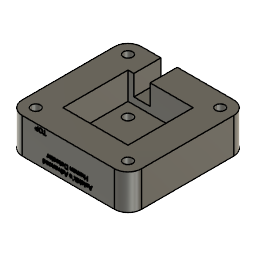
Sensor_Bottom (Autodesk Fusion 360 design; units mm, degrees)
part number: 2026-02-06-21-46-18-488
Autodesk Fusion 360 part; units mm, degrees
sketch "Sketch1" plane through (0, 0, 0) normal (0, 0, 1) x (1, 0, 0)
  line L0 (39, 33) -> (15, 33)
  line L1 (15, 33) -> (15, 9)
  line L2 (15, 9) -> (39, 9)
  line L3 (39, 9) -> (39, 33)
  circle A0 centre (44, 38) radius 1.7
  circle A1 centre (10, 38) radius 1.7
  circle A2 centre (44, 4) radius 1.7
  circle A3 centre (10, 4) radius 1.7
  line L4 (49, 43) -> (5, 43)
  line L5 (5, 43) -> (5, -1)
  line L6 (5, -1) -> (49, -1)
  line L7 (49, -1) -> (49, 43)
  circle A4 centre (44, 4) radius 3
  circle A5 centre (10, 4) radius 3
  circle A6 centre (44, 38) radius 3
  circle A7 centre (10, 38) radius 3
  dimension "d1" = 24
  dimension "d2" = 24
  dimension "d7" = 3.4
  dimension "d8" = 3.4
  dimension "d9" = 3.4
  dimension "d10" = 3.4
  dimension "d11" = 44
  dimension "d12" = 44
  dimension "d13" = 10
  dimension "d14" = 10
  dimension "d15" = 5
  dimension "d16" = 5
  dimension "d17" = 5
  dimension "d18" = 5
  dimension "d19" = 5
  dimension "d20" = 5
  dimension "d21" = 5
  dimension "d22" = 5
  dimension "d23" = 6
  dimension "d24" = 6
  dimension "d25" = 6
  dimension "d26" = 6
  constraint horizontal L0
  constraint vertical L1
  constraint horizontal L2
  constraint vertical L3
  constraint horizontal L4
  constraint vertical L5
  constraint horizontal L6
  constraint vertical L7
  constraint concentric A2 A4
  constraint concentric A3 A5
  constraint concentric A0 A6
  constraint concentric A1 A7
  measures "d1" distance of L0.start L0.end
  measures "d2" distance of L0.start L2.end
  measures "d7" diameter of A0
  measures "d8" diameter of A1 L3
  measures "d9" diameter of A2 L3
  measures "d10" diameter of A3
  measures "d11" distance of L4.start L4.end
  measures "d12" distance of L4.start L6.end
  measures "d13" distance of L3 L7
  measures "d14" distance of L0 L4
  measures "d15" distance of A2.centre L6
  measures "d16" distance of A2.centre L7
  measures "d17" distance of A3.centre L5
  measures "d18" distance of A3.centre L6
  measures "d19" distance of A0.centre L4
  measures "d20" distance of A0.centre L7
  measures "d21" distance of A1.centre L4
  measures "d22" distance of A1.centre L5
  measures "d23" diameter of A4 L3
  measures "d24" diameter of A5
  measures "d25" diameter of A6
  measures "d26" diameter of A7 L3
extrude "Extrude1" add sketch "Sketch1" along normal blind 9.9 from surface at 3.1 contours A4 | A5 | A6 | A7 makes body 1 at (12.9963, 37.8505, 9.7) makes body 2 at (46.9963, 3.8505, 9.7) makes body 3 at (41.0037, 37.8505, 9.7) makes body 4 at (12.9963, 3.8505, 9.7)
extrude "Extrude2" add sketch "Sketch1" along normal blind 13 contours L4 L5 L6 L7 bodies 1 2 3 4
extrude "Extrude3" add sketch "Sketch1" along normal blind 3 contours L0 L1 L2 L3 bodies 1
sketch "Sketch3" plane through (0, 0, 13) normal (0, 0, 1) x (-1, 0, 0)
  circle A0 centre (-10, -38) radius 1.7
  circle A1 centre (-10, -4) radius 1.7
  line L0 (-39, -33) -> (-39, -9)
  line L1 (-39, -9) -> (-15, -9)
  line L2 (-15, -9) -> (-15, -33)
  line L3 (-15, -33) -> (-39, -33)
  line L4 (-49, 1) -> (-49, -43)
  line L5 (-49, -43) -> (-5, -43)
  line L6 (-5, -43) -> (-5, 1)
  line L7 (-5, 1) -> (-49, 1)
  circle A2 centre (-44, -4) radius 1.7
  circle A3 centre (-44, -38) radius 1.7
  line L8 (-23.1675, -33) -> (-17.1675, -33)
  line L9 (-17.1675, -33) -> (-17.1675, -43)
  line L10 (-17.1675, -43) -> (-23.1675, -43)
  line L11 (-23.1675, -43) -> (-23.1675, -33)
  dimension "d35" = 6
  constraint horizontal L8
  constraint vertical L9
  constraint horizontal L10
  constraint vertical L11
  constraint coincident L5 L9.end
  constraint coincident L3 L8.start
  measures "d35" distance of L9 L11
extrude "Extrude4" cut sketch "Sketch3" against normal blind 7.5 contours L3 L5 L8 L9 L10 L11 bodies 1
fillet "Fillet1" radius 5 1 edges at (49, 43, 6.5) on bodies 1
fillet "Fillet1" radius 5 1 edges at (5, 43, 6.5) on bodies 1
fillet "Fillet1" radius 5 1 edges at (5, -1, 6.5) on bodies 1
fillet "Fillet1" radius 5 1 edges at (49, -1, 6.5) on bodies 1
sketch "Sketch4" plane through (0, 0, 3) normal (0, 0, 1) x (-1, 0, 0)
  line L0 (-39, -9) -> (-39, -33)
  line L1 (-39, -33) -> (-15, -33)
  line L2 (-15, -33) -> (-15, -9)
  line L3 (-15, -9) -> (-39, -9)
  circle A0 centre (-20, -28) radius 1.75
  circle A1 centre (-34, -14) radius 1.75
  dimension "d46" = 3.5
  dimension "d47" = 3.5
  dimension "d48" = 5
  dimension "d49" = 5
  dimension "d50" = 5
  dimension "d51" = 5
  measures "d46" diameter of A0
  measures "d47" diameter of A1
  measures "d48" distance of L1 A0.centre
  measures "d49" distance of L2 A0.centre
  measures "d50" distance of L3 A1.centre
  measures "d51" distance of L0 A1.centre
extrude "Extrude5" cut sketch "Sketch4" against normal blind 3 contours A0 | A1 bodies 1
sketch "Sketch5" plane through (0, -1, 0) normal (0, -1, 0) x (1, 0, 0)
  line L0 (44, 0) -> (44, 13)
  line L1 (44, 13) -> (10, 13)
  line L2 (10, 13) -> (10, 0)
  line L3 (10, 0) -> (44, 0)
  line L4 (36.4149, 5.1668) -> (16.996, 5.0019) construction
  line L5 (16.996, 5.0019) -> (17.0224, 1.8953) construction
  line L6 (17.0224, 1.8953) -> (36.4413, 2.0602) construction
  line L7 (36.4413, 2.0602) -> (36.4149, 5.1668) construction
  line L8 (23.2497, 12.5627) -> (10.2497, 12.5627) construction
  line L9 (10.2497, 12.5627) -> (10.2497, 10.5627) construction
  line L10 (10.2497, 10.5627) -> (23.2497, 10.5627) construction
  line L11 (23.2497, 10.5627) -> (23.2497, 12.5627) construction
  dimension "d54" = 1.5
  dimension "d56" = 1.5
  text T0 "Aoishik`s Advanced\nHuman Detector" font "Arial" height 1.5 align centre middle in box 19.4196 x 3.1067 at (36.4149, 5.1668) x (-0.999964, -0.008495) y (0.008495, -0.999964) spacing 1 kerned
  text T1 "TOP" font "Arial" height 1.5 align centre middle in box 13 x 2 at (23.2497, 12.5627) x (-1, 0) y (0, -1) spacing 1 kerned
extrude "Extrude6" cut sketch "Sketch5" against normal blind 0.8 text T0 T1 bodies 1
equation "d55 = 'Aoishik`s Advanced Human Detector'"
equation "d57 = 'TOP'"
